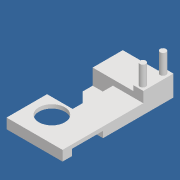
# Autodesk Inventor part: MotorHolder_Y
Saved by Autodesk Inventor 2020 (Build 240168000, 168)
## iProperties
Created: 2019-12-21
Part Number: MotorHolder_Y
Material: Generic
Document SubType Name: Modeling
Designer: Jack
Density: 1 g/cm^3
Appearance: Default
Author: Jack
Autodesk Inventor part; units mm, degrees
ref_plane "YZ Plane" through (0, 0, 0) normal (1, 0, 0) x (0, 1, 0)
ref_plane "XZ Plane" through (0, 0, 0) normal (0, 1, 0) x (-1, 0, 0)
ref_plane "XY Plane" through (0, 0, 0) normal (0, 0, 1) x (1, 0, 0)
sketch "Sketch1" plane through (0, 0, 0) normal (0, 1, 0) x (-1, 0, 0)
  line L0 (0, 0) -> (-24, 0)
  line L1 (-24, 0) -> (-24, -23.8)
  line L2 (-24, -23.8) -> (0, -23.8)
  line L3 (0, -23.8) -> (0, 0)
  dimension "d0" = 24
  dimension "d1" = 23.8
  constraints: 8 end point, 2 parallel, 1 horizontal, 1 perpendicular
  measures "d0" distance of L2.end L1.end
  measures "d1" distance of L1.end L0.end
extrude "Extrusion1" add sketch "Sketch1" along normal blind 8
sketch "Sketch3" plane through (0, 0, -23.8) normal (-1, 0, 0) x (0, 0, 1)
  line L0 (0, 8) -> (23.8, 8) projected
  line L1 (0, 8) -> (16, 8)
  line L2 (16, 8) -> (16, 5)
  line L3 (16, 5) -> (0, 5)
  line L4 (0, 5) -> (0, 8)
  point P0 (23.8, 0)
  dimension "d4" = 16
  dimension "d5" = 3
  constraints: 8 end point, 2 parallel, 1 horizontal, 1 perpendicular
  measures "d4" distance of L2.end L3.end
  measures "d5" distance of L1.end L2.end
extrude "Extrusion2" add sketch "Sketch3" along normal blind 8
sketch "Sketch4" plane through (0, 5, -23.8) normal (0, -1, 0) x (1, 0, 0)
  circle A0 centre (-4.3, 4) radius 2.35
  line L0 (0, 0) -> (0, 23.8) projected
  line L1 (0, 0) -> (-8, 0) projected
  dimension "d8" = 4.7
  dimension "d9" = 4.3
  dimension "d10" = 4
  constraints: 1 centre point
  measures "d8" diameter of A0
  measures "d9" distance from line of L0 A0.centre
  measures "d10" distance from line of L1 A0.centre
extrude "Extrusion3" add sketch "Sketch4" along normal blind 5
chamfer "Chamfer1" distance 8 angle 45 1 edges at (-8, 6.5, -7.8)
sketch "Sketch6" plane through (0, 0, 0) normal (0, 0, 1) x (1, 0, 0)
  line L0 (24, 8) -> (-8, 8) projected
  line L1 (24, 8) -> (8, 8)
  line L2 (8, 8) -> (8, 5)
  line L3 (8, 5) -> (24, 5)
  line L4 (24, 5) -> (24, 8)
  point P0 (0, 0)
  dimension "d18" = 16
  dimension "d19" = 3
  constraints: 8 end point, 2 parallel, 1 horizontal, 1 perpendicular
  measures "d18" distance of L3.end L2.end
  measures "d19" distance of L2.end L1.end
extrude "Extrusion4" add sketch "Sketch6" along normal blind 32
sketch "Sketch7" plane through (8, 5, 0) normal (0, -1, 0) x (1, 0, 0)
  line L0 (16, -23.8) -> (16, 32) projected
  line L1 (16, 32) -> (0, 32)
  line L2 (0, 32) -> (0, 24.4)
  line L3 (0, 24.4) -> (16, 24.4)
  line L4 (16, 24.4) -> (16, 32)
  point P0 (-8, 0)
  dimension "d22" = 16
  dimension "d23" = 7.6
  constraints: 8 end point, 2 parallel, 1 horizontal, 1 perpendicular
  measures "d22" distance of L3.end L2.end
  measures "d23" distance of L2.end L1.end
extrude "Extrusion5" add sketch "Sketch7" along normal blind 5
sketch "Sketch8" plane through (24, 0, -23.8) normal (0, 0, -1) x (-1, 0, 0)
  line L0 (0, 0) -> (0, 8) projected
  line L1 (24, 0) -> (24, 5) projected
  line L2 (0, 8) -> (24, 8)
  line L3 (24, 8) -> (24, 0)
  line L4 (24, 0) -> (0, 0)
  line L5 (0, 0) -> (0, 8)
  constraints: 8 end point, 2 parallel, 1 horizontal, 1 perpendicular
extrude "Extrusion6" add sketch "Sketch8" along normal blind 31.8
sketch "Sketch9" plane through (0, 8, 0) normal (0, 1, 0) x (1, 0, 0)
  circle A0 centre (19.7905, 51.6) radius 2.35
  circle A1 centre (19.8, 35.6) radius 2.35
  line L0 (0, 55.6) -> (24, 55.6) projected
  line L1 (0, 23.8) -> (0, 55.6) projected
  line L2 (0, 23.8) -> (-8, 23.8) projected
  point P0 (0, 0)
  dimension "d28" = 4.7
  dimension "d29" = 4.7
  dimension "d30" = 16
  dimension "d32" = 19.8
  dimension "d33" = 11.8
  constraints: 2 centre point
  measures "d28" diameter of A0
  measures "d29" diameter of A1
  measures "d30" distance of A0.centre A1.centre
  measures "d32" distance from line of L1 A1.centre
  measures "d33" distance from line of L2 A1.centre
sketch "Sketch10" plane through (0, 0, 0) normal (-1, 0, 0) x (0, 0, 1)
  line L0 (-23.8, 8) -> (-55.6, 8) projected
  line L1 (-55.6, 8) -> (-31.8, 8)
  line L2 (-31.8, 8) -> (-31.8, 0)
  line L3 (-31.8, 0) -> (-55.6, 0)
  line L4 (-55.6, 0) -> (-55.6, 8)
  point P0 (0, 0)
  dimension "d34" = 23.8
  dimension "d35" = 8
  constraints: 8 end point, 2 parallel, 1 horizontal, 1 perpendicular
  measures "d34" distance of L2.end L3.end
  measures "d35" distance of L1.end L2.end
extrude "Extrusion7" add sketch "Sketch10" along normal blind 16
sketch "Sketch11" plane through (0, 8, 0) normal (0, 1, 0) x (1, 0, 0)
  line L0 (-16, 55.6) -> (-16, 31.8) projected
  line L1 (24, 55.6) -> (-16, 55.6) projected
  line L2 (-16, 31.8) -> (24, 31.8)
  line L3 (24, 31.8) -> (24, 55.6)
  line L4 (24, 55.6) -> (-16, 55.6)
  line L5 (-16, 55.6) -> (-16, 31.8)
  point P0 (0, 0)
  constraints: 8 end point, 2 parallel, 1 horizontal, 1 perpendicular
extrude "Extrusion8" add sketch "Sketch11" along normal blind 4.4
extrude "Extrusion9" add sketch "Sketch9" along normal blind 24
sketch "Sketch12" plane through (0, 12.4, 0) normal (0, 1, 0) x (1, 0, 0)
  line L0 (24, 55.6) -> (16, 55.6)
  line L1 (16, 55.6) -> (16, 31.8)
  line L2 (16, 31.8) -> (24, 31.8)
  line L3 (24, 31.8) -> (24, 55.6)
  point P0 (0, 0)
  dimension "d42" = 8
  dimension "d43" = 23.8
  constraints: 8 end point, 2 parallel, 1 horizontal, 1 perpendicular
  measures "d42" distance of L2.end L1.end
  measures "d43" distance of L1.end L0.end
extrude "Extrusion10" add sketch "Sketch12" along normal blind 4
sketch "Sketch13" plane through (8, 5, 0) normal (-1, 0, 0) x (0, 0, 1)
  line L0 (0, 0) -> (0, 3) projected
  line L1 (0, 0) -> (24.4, 0) projected
  line L2 (24.4, 0) -> (24.4, -5) projected
  line L3 (32, -5) -> (24.4, -5) projected
  line L4 (32, 3) -> (32, -5) projected
  line L5 (0, 3) -> (32, 3) projected
  point P0 (0, -5)
extrude "Extrusion11" add sketch "Sketch13" along normal blind 28.2
sketch "Sketch14" plane through (0, 8, 0) normal (0, 1, 0) x (1, 0, 0)
  circle A0 centre (-4.2, -12.2) radius 10.25
  line L0 (-20.2, -32) -> (-20.2, 0) projected
  line L1 (0, 0) -> (-20.2, 0) projected
  line L2 (24, -32) -> (-20.2, -32) projected
  dimension "d48" = 20.5
  dimension "d49" = 16
  dimension "d51" = 19.8
  constraints: 1 centre point
  measures "d48" diameter of A0
  measures "d49" distance from line of L0 A0.centre
  measures "d51" distance from line of L2 A0.centre
extrude "Extrusion12" cut sketch "Sketch14" against normal blind 3
body "Solid1"
